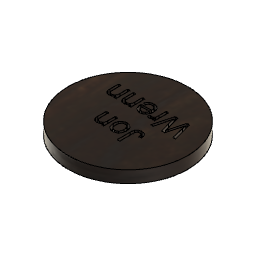
coaster v2 (Autodesk Fusion 360 design; units mm, degrees)
Autodesk Fusion 360 part; units mm, degrees
sketch "Sketch1" plane through (0, 0, 0) normal (0, 0, 1) x (1, 0, 0) in component "Coaster"
  circle A0 centre (0, 0) radius 25
  dimension "d1" = 50
  constraint coincident A0.centre origin
  measures "d1" diameter of A0
extrude "Extrude1" add sketch "Sketch1" along normal blind 5 in component "Coaster"
sketch "Sketch2" plane through (0, 0, 5) normal (0, 0, 1) x (-1, 0, 0) in component "Coaster"
  circle A0 centre (0, 0) radius 25
  line L0 (-13, -9) -> (12, -9) construction
  line L1 (12, -9) -> (12, 9) construction
  line L2 (12, 9) -> (-13, 9) construction
  line L3 (-13, 9) -> (-13, -9) construction
  dimension "d4" = 8
  text T0 "Jon Wrenn" font "Arial" height 8 align centre top in box 25 x 18 at (-13, -9) x (1, 0) y (0, 1) spacing 1 kerned
extrude "Extrude2" cut sketch "Sketch2" against normal blind 2 text T0 in component "Coaster"
component "Coaster" placed x (1, 0, 0) y (0, 1, 0) z (0, 0, 1) at (0, 0, 0)
